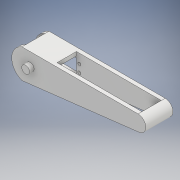
# Autodesk Inventor part: Tibia
Saved by Autodesk Inventor 2018 (Build 220112000, 112)
## iProperties
Created: 2020-03-07
Part Number: Tibia
Material: PVC, Unplasticized
Document SubType Name: Modeling
Designer: GonzaloDiaz
Density: 1.29 g/cm^3
Appearance: Smooth - White
Mass: 68.1388 g
Surface Area: 244.954 cm^2
Volume: 52.8208 cm^3
Author: GonzaloDiaz
Autodesk Inventor part; units mm, degrees
ref_plane "YZ Plane" through (0, 0, 0) normal (1, 0, 0) x (0, 1, 0)
ref_plane "XZ Plane" through (0, 0, 0) normal (0, 1, 0) x (-1, 0, 0)
sketch "Sketch1" plane through (0, 0, 0) normal (0, 1, 0) x (-1, 0, 0)
  line L0 (0, 0) -> (-150, 0)
  line L1 (-150, 0) -> (-150, -20) construction
  line L2 (-150, -20) -> (0, -37.6327)
  line L3 (0, -37.6327) -> (0, 0) construction
  arc A0 (-150, 0) -> (-150, -20) centre (-150, -10) ccw
  arc A1 (0, -37.6327) -> (0, 0) centre (-6.7783, -18.8163) ccw
  dimension "d0" = 150
  dimension "d1" = 20
  dimension "d3" = 20
  constraints: 8 end point, 4 point on circle, 2 centre point, 1 horizontal, 1 midpoint, 1 parallel, 1 vertical
  measures "d0" distance of L0.start L0.end
  measures "d1" distance of L0.end L1.end
  measures "d3" radius of A1
extrude "Extrusion1" add sketch "Sketch1" along normal blind 5
sketch "Sketch5" plane through (0, 5, 0) normal (0, 1, 0) x (1, 0, 0)
  line L0 (0, 7) -> (40.3, 7)
  line L1 (40.3, 7) -> (40.3, 27)
  line L2 (40.3, 27) -> (0, 27)
  line L3 (0, 27) -> (0, 7)
  line L4 (0, 0) -> (150, 0) projected
  arc A0 (0, 37.6327) -> (0, 0) centre (6.7783, 18.8163) ccw projected
  line L5 (0, 0) -> (0, 37.6327) construction
  dimension "d13" = 40.3
  dimension "d14" = 20
  dimension "d15" = 7
  dimension "d16" = 0
  constraints: 10 end point, 2 parallel, 1 horizontal, 1 perpendicular, 1 vertical
  measures "d13" distance of L2.end L1.end
  measures "d14" distance of L1.end L0.end
  measures "d15" distance between parallel lines of L4 L0
  measures "d16" distance between parallel lines of L5 L3
extrude "Extrusion3" cut sketch "Sketch5" against normal blind 5
ref_plane "Work Plane1" through (0, -12.5, 0) normal (0, -1, 0) x (1, 0, 0)
mirror "Mirror1" about plane through (0, -12.5, 0) normal (0, -1, 0) of "Extrusion1"
sketch "Sketch8" plane through (0, 0, 0) normal (0, 0, 1) x (1, 0, 0)
  line L0 (0, 0) -> (40.3, 0) projected
  line L1 (0, -25) -> (150, -25) projected
  line L2 (0, 0) -> (40.3767, 0)
  line L3 (40.3767, 0) -> (40.3767, -25)
  line L4 (40.3767, -25) -> (0, -25)
  line L5 (0, -25) -> (0, 0)
  constraints: 8 end point, 2 parallel, 1 horizontal, 1 perpendicular, 1 point on line
extrude "Extrusion4" add sketch "Sketch8" against normal blind 5
sketch "Sketch11" plane through (0, 5, 0) normal (0, 1, 0) x (1, 0, 0)
  circle A0 centre (-3.8458, 11.9975) radius 2
  circle A1 centre (-3.8458, 11.9975) radius 2 projected
  circle A2 centre (-3.8458, 21.9992) radius 2
  circle A3 centre (44.2605, 21.9992) radius 2
  circle A4 centre (-3.8458, 21.9992) radius 2 projected
  circle A5 centre (44.2605, 11.9975) radius 2 projected
  circle A6 centre (44.2605, 21.9992) radius 2 projected
  circle A7 centre (44.2605, 11.9975) radius 2
  point P0 (0, 0)
  constraints: 8 concentric, 4 centre point, 1 coincident, 3 other
extrude "Extrusion6" cut sketch "Sketch11" against normal blind 5
sketch "Sketch14" plane through (0, 0, -37.6327) normal (0.1167, 0, -0.9932) x (-0.9932, 0, -0.1167)
  line L0 (-151.0328, -25) -> (0, -25) projected
  line L1 (-4.3935, 0) -> (-44.3935, 0)
  line L2 (-44.3935, 0) -> (-44.3935, -25)
  line L3 (-44.3935, -25) -> (-4.3935, -25)
  line L4 (-4.3935, -25) -> (-4.3935, 0)
  dimension "d31" = 40
  constraints: 8 end point, 2 parallel, 1 horizontal, 1 perpendicular, 1 point on line
  measures "d31" distance of L3.end L2.end
extrude "Extrusion7" add sketch "Sketch14" against normal blind 5
sketch "Sketch17" plane through (0, 5, 0) normal (0, 1, 0) x (1, 0, 0)
  arc A0 (150, 0) -> (150, 20) centre (150, 10) ccw projected
  line L0 (150, 20) -> (44.0899, 32.4499) projected
  line L1 (150, 0) -> (150, 20)
  point P0 (0, 0)
  constraints: 2 end point, 1 vertical
extrude "Extrusion10" add sketch "Sketch17" against normal up to surface (35 mm away)
sketch "Sketch18" plane through (0, -30, 0) normal (0, -1, 0) x (1, 0, 0)
  circle A0 centre (10.7396, -16.9983) radius 5
  circle A1 centre (10.7396, -16.9983) radius 2.9 projected
  point P0 (0, 0)
  dimension "d42" = 10
  constraints: 1 centre point, 1 concentric
  measures "d42" diameter of A0
extrude "Extrusion11" add sketch "Sketch18" along normal blind 6 contours A0 | A1
body "Solid1"
